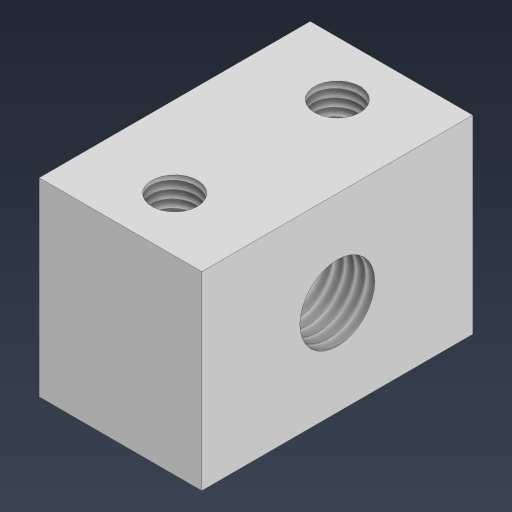
# Autodesk Inventor part: 3D Model
Saved by Autodesk Inventor 2024 (Build 280153000, 153)
## iProperties
Created: 2024-03-07
Part Number: 3D Model
Material: Genérico
Document SubType Name: Modeling
Designer: Administrator
Density: 1 g/cm^3
Appearance: Padrão
Author: Administrator
Autodesk Inventor part; units mm, degrees
ref_plane "YZ Plane" through (0, 0, 0) normal (1, 0, 0) x (0, 1, 0)
ref_plane "XZ Plane" through (0, 0, 0) normal (0, 1, 0) x (-1, 0, 0)
ref_plane "XY Plane" through (0, 0, 0) normal (0, 0, 1) x (1, 0, 0)
sketch "Esboço1" plane through (0, 0, 0) normal (0, 1, 0) x (-1, 0, 0)
  line L0 (15, -25) -> (-15, -25)
  line L1 (-15, -25) -> (-15, 25)
  line L2 (-15, 25) -> (15, 25)
  line L3 (15, 25) -> (15, -25)
  line L4 (15, -25) -> (-15, 25) construction
  line L5 (-15, -25) -> (15, 25) construction
  point P0 (0, 0)
  dimension "d0" = 30
  dimension "d1" = 50
  constraints: 12 end point, 2 midpoint, 2 parallel, 1 horizontal, 1 perpendicular
  measures "d0" distance of L1.end L2.end
  measures "d1" distance of L0.end L1.end
extrude "Extrusão1" add sketch "Esboço1" along normal blind 35
sketch "Esboço3" plane through (0, 35, 0) normal (0, 1, 0) x (1, 0, 0)
  line L0 (-15, -25) -> (15, -25) projected
  line L1 (-15, 25) -> (-15, -25) projected
  point P0 (0, 0)
  point P1 (0, -15)
  dimension "d4" = 10
  dimension "d5" = 15
  measures "d4" distance from line of L0 point (0, -15)
  measures "d5" distance from line of L1 point (0, -15)
hole "Furo1" at (0, 35, 15) direction (0, -1, 0) diameter 8.376 depth 27.3 tip angle 118 thread size "M10x1.5" class "6H" standard "ISO Metric profile"
sketch "Esboço4" plane through (0, 35, 0) normal (0, 1, 0) x (1, 0, 0)
  line L0 (15, 25) -> (-15, 25) projected
  line L1 (-15, 25) -> (-15, -25) projected
  point P0 (0, 0)
  point P1 (0, 15)
  dimension "d13" = 10
  dimension "d14" = 15
  measures "d13" distance from line of L0 point (0, 15)
  measures "d14" distance from line of L1 point (0, 15)
hole "Furo2" at (0, 35, -15) direction (0, -1, 0) diameter 8.376 end through all thread size "M10x1.5" class "6H" standard "ISO Metric profile"
sketch "Esboço5" plane through (15, 0, 25) normal (1, 0, 0) x (0, 0, -1)
  line L0 (0, 0) -> (0, 35) projected
  line L1 (0, 35) -> (50, 35) projected
  point P0 (25, 0)
  point P1 (25, 17.5)
  dimension "d22" = 25
  dimension "d23" = 17.5
  measures "d22" distance from line of L0 point (25, 17.5)
  measures "d23" distance from line of L1 point (25, 17.5)
hole "Furo3" at (15, 17.5, 0) direction (-1, 0, 0) diameter 13.835 end through all thread size "M16x2" class "6H" standard "ISO Metric profile"
